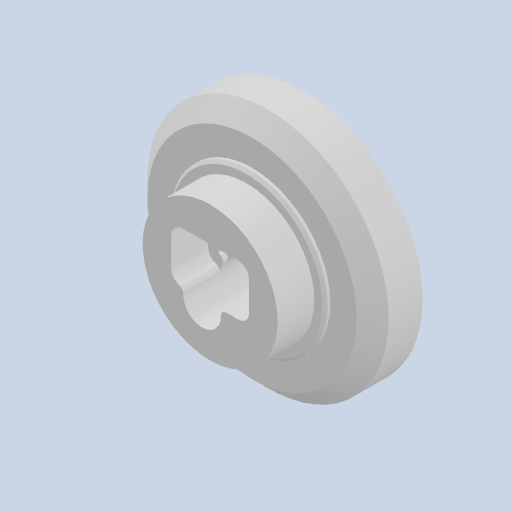
# Autodesk Inventor part: wheel_fixator
Saved by Autodesk Inventor 2022 (Build 260153000, 153)
## iProperties
Created: 2024-09-10
Part Number: wheel_fixator
Material: Типовые
Document SubType Name: Modeling
Designer: Andrey
Density: 1 g/cm^3
Appearance: По умолчанию
Author: Andrey
Autodesk Inventor part; units mm, degrees
ref_plane "YZ Plane" through (0, 0, 0) normal (1, 0, 0) x (0, 1, 0)
ref_plane "XZ Plane" through (0, 0, 0) normal (0, 1, 0) x (-1, 0, 0)
ref_plane "XY Plane" through (0, 0, 0) normal (0, 0, 1) x (1, 0, 0)
sketch "Эскиз1" plane through (0, 0, 0) normal (0, 0, 1) x (1, 0, 0)
  circle A0 centre (0, 0) radius 22.5
  dimension "d0" = 45
  constraints: 1 centre point, 1 coincident
  measures "d0" diameter of A0
extrude "Выдавливание1" add sketch "Эскиз1" along normal blind 9.295
sketch "Эскиз2" plane through (0, 0, 9.295) normal (0, 0, 1) x (1, 0, 0)
  circle A0 centre (0, 0) radius 12.6
  dimension "d3" = 25.2
  constraints: 1 centre point, 1 coincident
  measures "d3" diameter of A0
extrude "Выдавливание2" add sketch "Эскиз2" along normal blind 7.8
sketch "Эскиз3" plane through (0, 0, 9.295) normal (0, 0, 1) x (1, 0, 0)
  circle A0 centre (0, 0) radius 12.6 projected
  circle A1 centre (0, 0) radius 22.5 projected
  circle A2 centre (0, 0) radius 14.6
  dimension "d6" = 2
  constraints: 1 centre point
  measures "d6" radial gap between concentric circles of A0 A2
extrude "Выдавливание3" add sketch "Эскиз3" along normal blind 1 contours A2
chamfer "Фаска1" distance 0.5 angle 45 1 edges at (-14.6, 0, 10.295)
sketch "Эскиз4" plane through (0, 0, 17.095) normal (0, 0, 1) x (1, 0, 0)
  line L0 (0, 0) -> (0, -1.1)
  line L1 (5, -1.1) -> (-5, -1.1)
  line L2 (-5, -1.1) -> (-5, 3.9)
  line L3 (-5, 3.9) -> (5, 3.9)
  line L4 (5, 3.9) -> (5, -1.1)
  circle A0 centre (0, 0) radius 12.6 projected
  line L5 (-5.25, -1.35) -> (5.25, -1.35)
  line L6 (5.25, -1.35) -> (5.25, 4.15)
  line L7 (5.25, 4.15) -> (-5.25, 4.15)
  line L8 (-5.25, 4.15) -> (-5.25, -1.35)
  dimension "d45" = 1.1
  dimension "d46" = 10
  dimension "d47" = 5
  dimension "d48" = 0.25
  constraints: 18 end point, 4 parallel, 2 perpendicular, 1 coincident, 1 horizontal, 1 midpoint, 1 vertical, 3 other
  measures "d45" distance of L0.end L0.start
  measures "d46" distance of L2.end L3.end
  measures "d47" distance of L1.end L2.end
  measures "d48" distance between parallel lines of L1 L5
extrude "Выдавливание4" cut sketch "Эскиз4" against normal blind 7.8 contours L1 L2 L3 L4 | L8 L7 L6 L5
sketch "Эскиз5" plane through (0, 0, 0) normal (0, 0, -1) x (-1, 0, 0)
  circle A0 centre (13.4441, 11.2809) radius 1.5 projected
  circle A1 centre (0, 17.55) radius 1.5 projected
  circle A2 centre (-13.4441, 11.2809) radius 1.5 projected
  circle A3 centre (13.4441, 11.2809) radius 2.1
  circle A4 centre (0, 17.55) radius 2.1
  circle A5 centre (-13.4441, 11.2809) radius 2.1
  point P0 (0, 0)
  dimension "d16" = 4.2
  dimension "d17" = 4.2
  dimension "d18" = 4.2
  constraints: 3 centre point, 3 coincident
  measures "d16" diameter of A3
  measures "d17" diameter of A4
  measures "d18" diameter of A5
extrude "Выдавливание5" cut sketch "Эскиз5" against normal blind 7.8 contours A0 | A1 | A2 | A3 | A4 | A5
sketch "Эскиз6" plane through (0, 0, 17.095) normal (0, 0, 1) x (1, 0, 0)
  circle A0 centre (-1.5, -4.5) radius 1.5 projected
  circle A1 centre (-1.5, -4.5) radius 3.5
  point P0 (0, 0)
  dimension "d21" = 7
  constraints: 1 centre point, 1 coincident
  measures "d21" diameter of A1
extrude "Выдавливание6" cut sketch "Эскиз6" against normal blind 13 contours A0 | A1
sketch "Эскиз7" plane through (-1.5, -4.5, 4.095) normal (0, 0, 1) x (1, 0, 0)
  circle A0 centre (0, 0) radius 3.5 projected
  circle A1 centre (0, 0) radius 1.6
  point P0 (1.5, 4.5)
  dimension "d24" = 3.2
  constraints: 1 centre point, 1 coincident
  measures "d24" diameter of A1
extrude "Выдавливание7" cut sketch "Эскиз7" against normal blind 13 contours A1
chamfer "Фаска2" distance 3 angle 45 1 edges at (-22.5, 0, 9.295)
sketch "Эскиз10" plane through (0, 0, 17.095) normal (0, 0, 1) x (1, 0, 0)
  arc A0 (0.0256, -1.35) -> (-3.0256, -1.35) centre (-1.5, -4.5) ccw projected
  line L0 (5.25, -1.35) -> (0.0256, -1.35) projected
  line L1 (5.25, 4.15) -> (5.25, -1.35) projected
  line L2 (-5.25, 4.15) -> (5.25, 4.15) projected
  line L3 (-5.25, -1.35) -> (-5.25, 4.15) projected
  line L4 (-3.0256, -1.35) -> (-5.25, -1.35) projected
  circle A1 centre (0, 0) radius 12.6 projected
  arc A2 (-3.0256, -1.35) -> (0.0256, -1.35) centre (-1.5, -4.5) ccw projected
  line L5 (-3.0256, -1.35) -> (-5.25, -1.35) projected
  line L6 (-5.25, -1.35) -> (-5.25, 4.15) projected
  line L7 (-5.25, 4.15) -> (5.25, 4.15) projected
  line L8 (5.25, 4.15) -> (5.25, -1.35) projected
  line L9 (5.25, -1.35) -> (0.0256, -1.35) projected
  arc A3 (-0.5369, -3.35) -> (-2.4631, -3.35) centre (-1.5, -4.5) ccw
  line L10 (-2.4631, -3.35) -> (-7.25, -3.35)
  line L11 (-7.25, -3.35) -> (-7.25, 6.15)
  line L12 (-7.25, 6.15) -> (7.25, 6.15)
  line L13 (7.25, 6.15) -> (7.25, -3.35)
  line L14 (7.25, -3.35) -> (-0.5369, -3.35)
  point P0 (-4.8057, -3.35)
  point P1 (-3.0256, -1.35)
  point P2 (0.0256, -1.35)
  point P3 (1.8057, -3.35)
  dimension "d49" = 2
  constraints: 10 end point, 2 point on circle, 1 centre point, 5 other
  measures "d49" distance between parallel lines of L0 L14
extrude "Выдавливание10" cut sketch "Эскиз10" against normal blind 6.85 contours L0 L1 L2 L3 L4 A2 L10 L11 L12 L13 L14
fillet "Сопряжение3" radius 2 4 edges at (7.25, -3.35, 13.67) (-7.25, -3.35, 13.67) (-7.25, 6.15, 13.67) (7.25, 6.15, 13.67)
fillet "Сопряжение4" radius 1 4 edges at (1.8057, -3.35, 13.67) (-4.8057, -3.35, 13.67) (0.0256, -1.35, 9.77) (-3.0256, -1.35, 9.77)
